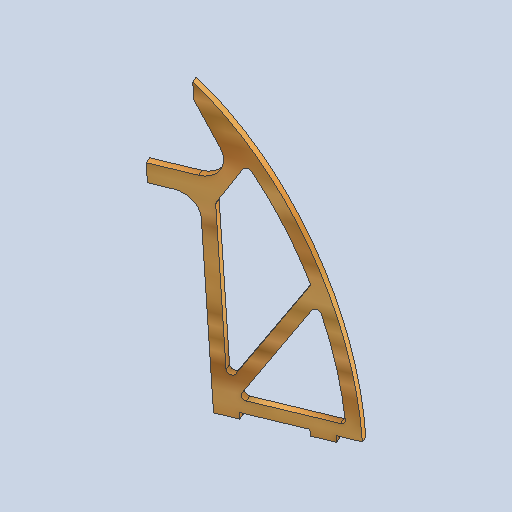
# Autodesk Inventor part: aux_nose_bottom
Saved by Autodesk Inventor 2022 (Build 260153070, 153G)
## iProperties
Created: 2021-04-25
Part Number: aux_nose_bottom
Material: Plywood, Sheathing, Glazed
Document SubType Name: Modeling
Designer: kardo
Density: 0.75 g/cm^3
Appearance: Plywood - New(2)
Mass: 1.82443 g
Surface Area: 34.7762 cm^2
Volume: 2.43258 cm^3
Author: kardo
Autodesk Inventor part; units mm, degrees
ref_plane "YZ Plane" through (0, 0, 0) normal (1, 0, 0) x (0, 1, 0)
ref_plane "XZ Plane" through (0, 0, 0) normal (0, 1, 0) x (-1, 0, 0)
ref_plane "XY Plane" through (0, 0, 0) normal (0, 0, 1) x (1, 0, 0)
derived "frame_outline.ipt"
sketch "aux_node_bottom" plane through (81, 0, 19.8753) normal (-0.3533007, 0.0652579, -0.933231) x (0.9352244, 0, -0.3540554)
  line L0 (52.1093, -130.6087) -> (0.0129, -129.3216)
  line L1 (0.0129, -129.3216) -> (-2.607, -235.3661)
  spline S0 degree 3 poles (52.9091, -130.6284) (51.7644, -176.9604) (26.8076, -226.1581) (-5.8676, -237.5063) knots 0 0 0 0 1 1 1 1
  spline S1 degree 3 poles (52.1093, -130.6087) (52.018, -134.3054) (51.5303, -141.7374) (50.1989, -151.0178) (48.3571, -160.2111) (46.4879, -167.4644) (43.6878, -176.3245) (41.0896, -183.2155) (37.4257, -191.5035) (34.1746, -197.8412) (29.7429, -205.3183) (25.9163, -210.912) (20.8144, -217.34) (16.4914, -221.9996) (10.8197, -227.1425) (4.8969, -231.565) (-0.0729, -234.2536) (-2.607, -235.3661) knots 0 0 0 0 0.080261 0.160521 0.200651 0.280912 0.321042 0.401303 0.441433 0.521694 0.561824 0.642085 0.682215 0.762475 0.802606 0.882866 0.963127 0.963127 0.963127 0.963127
  point P0 (-68.7162, 3.0845)
  point P1 (-2.6288, -236.2478)
  point P2 (-1.6454, -196.4445)
extrude "Extrusion1" add sketch "aux_node_bottom" against normal blind 2
sketch "Sketch2" plane through (84.7066, 128.9155, 29.6298) normal (0.3533007, -0.0652579, 0.933231) x (0.9355098, 0.024645, -0.3524401)
  line L0 (0, 0) -> (52.1123, 0) projected
  line L1 (0, 106.0768) -> (0, 0) projected
  line L2 (45.3377, 0) -> (45.3377, -2)
  line L3 (45.3377, -2) -> (38.5631, -2)
  line L4 (38.5631, -2) -> (38.5631, 0)
  line L5 (20.3238, 0) -> (20.3238, -2)
  line L6 (20.3238, -2) -> (13.5492, -2)
  line L7 (13.5492, -2) -> (13.5492, 0)
  point P0 (-71.9782, -130.6683)
  dimension "d3" = 52.1123
  dimension "d4" = 6.7746
  dimension "d5" = 6.7746
  dimension "d6" = 6.7746
  dimension "d7" = 13.5492
  dimension "d8" = 2
  constraints: 12 end point, 4 perpendicular, 4 point on line, 1 collinear, 1 parallel, 1 other
  measures "d3" distance of L0.start L0.end
  measures "d4" distance of L2.end L3.end
  measures "d5" distance of L5.end L6.end
  measures "d6" distance from line of L0.end L2
  measures "d7" distance of L0.start L7.end
  measures "d8" distance of L3.end L4.end
extrude "fins" add sketch "Sketch2" against normal up to surface (2 mm away)
sketch "Sketch3" plane through (84.7066, 128.9155, 29.6298) normal (0.3533007, -0.0652579, 0.933231) x (0.9355098, 0.024645, -0.3524401)
  line L0 (13.5492, 0) -> (13.5492, -2) projected
  line L1 (0, 106.0768) -> (0, 0) projected
  spline S0 degree 3 poles (52.1123, 0) (52.1123, 3.6978) (51.8083, 11.1397) (50.7066, 20.45) (49.0924, 29.6861) (47.4029, 36.9833) (44.8225, 45.9099) (42.3952, 52.863) (38.9372, 61.2389) (35.8436, 67.655) (31.5979, 75.2392) (27.9106, 80.9257) (22.9691, 87.4778) (18.7625, 92.2427) (13.2194, 97.5241) (7.4077, 102.0915) (2.5059, 104.9021) (0, 106.0768) knots 0 0 0 0 0.083333 0.166667 0.208333 0.291667 0.333333 0.416667 0.458333 0.541667 0.583333 0.666667 0.708333 0.791667 0.833333 0.916667 1 1 1 1 projected
  line L2 (13.5492, 0) -> (0, 0) projected
  line L3 (13.5492, 0) -> (13.5492, 56.3688)
  line L4 (0, 63.1434) -> (6.7746, 63.1434)
  line L5 (0, 69.1434) -> (13.5492, 69.1434)
  arc A0 (13.5492, 56.3688) -> (6.7746, 63.1434) centre (6.7746, 56.3688) ccw
  line L6 (17.5492, 4) -> (48.0519, 4)
  line L7 (20.3238, 0) -> (38.5631, 0) projected
  arc A1 (13.5492, 69.1434) -> (19.7046, 78.9671) centre (13.5492, 75.9837) ccw
  line L8 (19.7046, 78.9671) -> (13.5492, 91.6672)
  line L9 (19.7046, 78.9671) -> (23.1076, 80.6165) construction
  line L10 (6.7746, 56.3688) -> (13.5492, 56.3688) construction
  line L11 (17.5492, 4) -> (17.5492, 61.9513)
  line L12 (17.5492, 61.9513) -> (26.3223, 75.9527)
  line L13 (13.5492, 75.9837) -> (19.3457, 72.3517) construction
  line L14 (19.3457, 72.3517) -> (22.7352, 70.2279) construction
  line L15 (13.5492, 91.6672) -> (13.5492, 97.0919)
  line L16 (13.5492, 69.1434) -> (19.3457, 72.3517) construction
  line L17 (19.3457, 72.3517) -> (19.7046, 78.9671) construction
  line L18 (17.5492, 4) -> (41.9454, 41.4133) construction
  line L19 (19.9368, 4) -> (42.6763, 38.8725)
  line L20 (17.5492, 7.6616) -> (41.1817, 43.9037)
  line L21 (26.3223, 75.9527) -> (41.9454, 41.4133) construction
  line L22 (41.9454, 41.4133) -> (48.0519, 4) construction
  line L23 (0, 67.1434) -> (0, 65.1434)
  line L24 (0, 65.1434) -> (0, 63.1434)
  line L25 (0, 67.1434) -> (0, 69.1434)
  spline S1 degree 5 poles (48.0519, 4) (47.8793, 9.74) (47.4018, 15.4709) (46.642, 21.1718) (44.4614, 33.154) (41.0918, 44.8611) (38.9875, 50.942) (34.3298, 62.3301) (28.376, 73.0944) (25.2237, 78.0498) (20.9861, 83.7841) (16.1825, 89.0189) (15.3229, 89.9198) (14.4453, 90.8031) (13.5492, 91.6672) knots 0 0 0 0 0 0 0.298027 0.298027 0.298027 0.631351 0.631351 0.631351 0.935395 0.935395 0.935395 1 1 1 1 1 1
  point P0 (-71.9782, -130.6683)
  dimension "d15" = 4
  dimension "d14" = 4
  dimension "d16" = 6
  dimension "d18" = 106.0768
  dimension "d20" = 15
  dimension "d21" = 4
  dimension "d22" = 4
  dimension "d23" = 4
  dimension "d27" = 2
  constraints: 44 end point, 8 point on line, 5 parallel, 5 point on circle, 4 equal length, 4 perpendicular, 4 tangent, 2 centre point, 2 collinear, 11 other
  measures "d14" distance between parallel lines of L7 L6
  measures "d16" distance between parallel lines of L5 L4
  measures "d18" distance of L1.start L1.end
  measures "d21" distance between parallel lines of L3 L11
  measures "d22" distance of L13.end L14.end
  measures "d23" distance between parallel lines of L20 L19
  measures "d27" distance of L23.start L23.end
extrude "Extrusion3" cut sketch "Sketch3" against normal through all both and the other way through all contours S0 L15 L8 A1 L5 L1 | L4 A0 L3 L2 L1 | L19 S1 L6 | L11 L12 S1 L20
fillet "Fillet1" radius 1.3333 6 edges at (103.0044, 133.4623, 21.9491) (100.7708, 191.2136, 26.8331) (108.9781, 205.3971, 24.7178) (124.2774, 168.8103, 16.3674) (129.3063, 134.1552, 12.0402) (100.7708, 137.0562, 23.046)
equation "\"d1\" = bulkhead_thickness"
equation "\"d4\" = 0.13 * d3"
equation "\"d5\" = d4"
equation "\"d6\" = d4"
equation "\"d7\" = 2 * d5"
equation "\"d8\" = bulkhead_thickness"
equation "\"d15\" = inset"
equation "\"d14\" = inset"
equation "\"d16\" = 3 * bulkhead_thickness"
equation "\"d21\" = inset"
equation "\"d22\" = inset"
equation "\"d23\" = inset"
equation "\"d27\" = bulkhead_thickness"
equation "\"d26\" = 0.333333 * inset"
equation "\"bulkhead_thickness\" = 2"
equation "\"inset\" = 4"
body "Solid1"
